Autodesk Fusion 360 part; units mm, degrees
(part 2 of 3)
  line L411 (91.783, -75.7587) -> (82.1412, -64.2681)
  line L412 (106.6546, -43.6989) -> (116.2964, -55.1895)
  line L413 (116.2964, -55.1895) -> (104.8058, -64.8313)
  line L414 (104.8058, -64.8313) -> (95.164, -53.3407)
  line L415 (95.164, -53.3407) -> (106.6546, -43.6989)
  line L416 (6.4022, 0.3248) -> (20.3282, -16.2717)
  line L417 (20.3282, -16.2717) -> (18.7961, -17.5572)
  line L418 (18.7961, -17.5572) -> (30.3663, -31.346)
  line L419 (30.3663, -31.346) -> (25.77, -35.2028)
  line L420 (25.77, -35.2028) -> (41.1969, -53.5878)
  line L421 (41.1969, -53.5878) -> (44.2611, -51.0167)
  line L422 (44.2611, -51.0167) -> (55.8313, -64.8055)
  line L423 (55.8313, -64.8055) -> (65.0238, -57.092)
  line L424 (65.0238, -57.092) -> (76.594, -70.8808)
  line L425 (76.594, -70.8808) -> (79.6582, -68.3097)
  line L426 (79.6582, -68.3097) -> (91.2284, -82.0985)
  line L427 (91.2284, -82.0985) -> (135.6589, -44.8168)
  line L428 (135.6589, -44.8168) -> (120.232, -26.4317)
  line L429 (120.232, -26.4317) -> (117.1679, -29.0029)
  line L430 (117.1679, -29.0029) -> (105.5977, -15.2141)
  line L431 (105.5977, -15.2141) -> (96.4051, -22.9275)
  line L432 (96.4051, -22.9275) -> (84.835, -9.1387)
  line L433 (84.835, -9.1387) -> (81.7708, -11.7099)
  line L434 (81.7708, -11.7099) -> (74.0573, -2.5173)
  line L435 (74.0573, -2.5173) -> (78.6536, 1.3394)
  line L436 (78.6536, 1.3394) -> (74.1541, 6.7017)
  line L437 (74.1541, 6.7017) -> (91.7731, 21.4858)
  line L438 (91.7731, 21.4858) -> (56.8473, 63.1088)
  line L439 (56.8473, 63.1088) -> (16.3349, 82)
  line L440 (16.3349, 82) -> (-38, 82)
  line L441 (-38, 82) -> (-38, 59)
  line L442 (-38, 59) -> (-45, 59)
  line L443 (-45, 59) -> (-45, 53)
  line L444 (-45, 53) -> (-57, 53)
  line L445 (-57, 53) -> (-57, 57)
  line L446 (-57, 57) -> (-75, 57)
  line L447 (-75, 57) -> (-75, 69)
  line L448 (-75, 69) -> (-93, 69)
  line L449 (-93, 69) -> (-93, 73)
  line L450 (-93, 73) -> (-117, 73)
  line L451 (-117, 73) -> (-117, 15)
  line L452 (-117, 15) -> (-99, 15)
  line L453 (-99, 15) -> (-99, 11)
  line L454 (-99, 11) -> (-81, 11)
  line L455 (-81, 11) -> (-81, -1)
  line L456 (-81, -1) -> (-63, -1)
  line L457 (-63, -1) -> (-63, -5)
  line L458 (-63, -5) -> (-39, -5)
  line L459 (-39, -5) -> (-39, 1)
  line L460 (-39, 1) -> (-21, 1)
  line L461 (-21, 1) -> (-21, 3)
  line L462 (-21, 3) -> (0.6651, 3)
  line L463 (0.6651, 3) -> (6.4022, 0.3248)
  dimension "d150" = -0.5
  dimension "d151" = -3
extrude "Extrude16" add sketch "Sketch15" along normal blind 1 contours L160 L161 L162 L163 L164 L165 L166 L167 L168 L169 L170 L171 L172 L173 L174 L175 L176 L177 L178 L179 L180 L181 L182 L183 L184 L185 L186 L187 L188 L189 L190 L191 L192 L193 L194 L195 L196 L197 L198 L199 L200 L201 L202 L203 L204 L205 L206 L207 | L292 L293 L294 L295 L296 L297 L298 L299 L300 L301 L302 L303 L304 L305 L306 L307 L308 L309 L310 L311 L312 L313 L314 L315 L316 L317 L318 L319 L320 L321 L322 L323 L324 L325 L326 L327 L328 L329 L330 L331 L332 L333 L334 L335 L336 L337 L338 L339 | L416 L417 L418 L419 L420 L421 L422 L423 L424 L425 L426 L427 L428 L429 L430 L431 L432 L433 L434 L435 L436 L437 L438 L439 L440 L441 L442 L443 L444 L445 L446 L447 L448 L449 L450 L451 L452 L453 L454 L455 L456 L457 L458 L459 L460 L461 L462 L463
sketch "Sketch16" plane through (0, 2.3, 0) normal (0, 1, 0) x (-1, 0, 0)
  line L0 (62.672, 13.3847) -> (72.3139, 1.894)
  line L1 (72.3139, 1.894) -> (60.8232, -7.7478)
  line L2 (60.8232, -7.7478) -> (51.1814, 3.7429)
  line L3 (51.1814, 3.7429) -> (62.672, 13.3847)
  line L4 (92.0203, -32.4812) -> (101.6621, -43.9719)
  line L5 (101.6621, -43.9719) -> (90.1714, -53.6137)
  line L6 (90.1714, -53.6137) -> (80.5296, -42.123)
  line L7 (80.5296, -42.123) -> (92.0203, -32.4812)
  line L8 (32.1098, -35.7574) -> (43.6004, -26.1156)
  line L9 (43.6004, -26.1156) -> (53.2423, -37.6063)
  line L10 (53.2423, -37.6063) -> (41.7516, -47.2481)
  line L11 (41.7516, -47.2481) -> (32.1098, -35.7574)
  line L12 (-58.5, 33.5) -> (-58.5, 48.5)
  line L13 (-58.5, 48.5) -> (-43.5, 48.5)
  line L14 (-43.5, 48.5) -> (-43.5, 33.5)
  line L15 (-43.5, 33.5) -> (-58.5, 33.5)
  line L16 (49.6493, 2.4573) -> (59.2911, -9.0334)
  line L17 (59.2911, -9.0334) -> (47.8004, -18.6752)
  line L18 (47.8004, -18.6752) -> (38.1586, -7.1845)
  line L19 (38.1586, -7.1845) -> (49.6493, 2.4573)
  line L20 (39.6112, 17.5317) -> (49.253, 6.041)
  line L21 (49.253, 6.041) -> (37.7623, -3.6008)
  line L22 (37.7623, -3.6008) -> (28.1205, 7.8899)
  line L23 (28.1205, 7.8899) -> (39.6112, 17.5317)
  line L24 (-40.5, 37.5) -> (-25.5, 37.5)
  line L25 (-25.5, 37.5) -> (-25.5, 22.5)
  line L26 (-25.5, 22.5) -> (-40.5, 22.5)
  line L27 (-40.5, 22.5) -> (-40.5, 37.5)
  line L28 (77.1487, -64.5411) -> (67.5068, -53.0504)
  line L29 (67.5068, -53.0504) -> (78.9975, -43.4086)
  line L30 (78.9975, -43.4086) -> (88.6393, -54.8993)
  line L31 (88.6393, -54.8993) -> (77.1487, -64.5411)
  line L32 (72.7896, -25.1203) -> (84.2803, -15.4785)
  line L33 (84.2803, -15.4785) -> (93.9221, -26.9691)
  line L34 (93.9221, -26.9691) -> (82.4315, -36.611)
  line L35 (82.4315, -36.611) -> (72.7896, -25.1203)
  line L36 (73.9427, 12.3986) -> (64.3009, 23.8893)
  line L37 (64.3009, 23.8893) -> (75.7916, 33.5311)
  line L38 (75.7916, 33.5311) -> (85.4334, 22.0405)
  line L39 (85.4334, 22.0405) -> (73.9427, 12.3986)
  line L40 (-58.5, 14.5) -> (-43.5, 14.5)
  line L41 (-43.5, 14.5) -> (-43.5, -0.5)
  line L42 (-43.5, -0.5) -> (-58.5, -0.5)
  line L43 (-58.5, -0.5) -> (-58.5, 14.5)
  line L44 (36.2303, -4.8864) -> (24.7396, -14.5282)
  line L45 (24.7396, -14.5282) -> (15.0978, -3.0375)
  line L46 (15.0978, -3.0375) -> (26.5884, 6.6043)
  line L47 (26.5884, 6.6043) -> (36.2303, -4.8864)
  line L48 (-79.5, 49.5) -> (-94.5, 49.5)
  line L49 (-94.5, 49.5) -> (-94.5, 64.5)
  line L50 (-94.5, 64.5) -> (-79.5, 64.5)
  line L51 (-79.5, 64.5) -> (-79.5, 49.5)
  line L52 (-94.5, 30.5) -> (-79.5, 30.5)
  line L53 (-79.5, 30.5) -> (-79.5, 15.5)
  line L54 (-79.5, 15.5) -> (-94.5, 15.5)
  line L55 (-94.5, 15.5) -> (-94.5, 30.5)
  line L56 (45.1325, -24.83) -> (56.6232, -15.1882)
  line L57 (56.6232, -15.1882) -> (66.265, -26.6789)
  line L58 (66.265, -26.6789) -> (54.7743, -36.3207)
  line L59 (54.7743, -36.3207) -> (45.1325, -24.83)
  line L60 (-112.5, 51.5) -> (-97.5, 51.5)
  line L61 (-97.5, 51.5) -> (-97.5, 36.5)
  line L62 (-97.5, 36.5) -> (-112.5, 36.5)
  line L63 (-112.5, 36.5) -> (-112.5, 51.5)
  line L64 (-22.5, 39.5) -> (-7.5, 39.5)
  line L65 (-7.5, 39.5) -> (-7.5, 24.5)
  line L66 (-7.5, 24.5) -> (-22.5, 24.5)
  line L67 (-22.5, 24.5) -> (-22.5, 39.5)
  line L68 (105.043, -21.5538) -> (114.6848, -33.0445)
  line L69 (114.6848, -33.0445) -> (103.1942, -42.6863)
  line L70 (103.1942, -42.6863) -> (93.5524, -31.1956)
  line L71 (93.5524, -31.1956) -> (105.043, -21.5538)
  line L72 (-15.5, 62.5) -> (-15.5, 77.5)
  line L73 (-15.5, 77.5) -> (-0.5, 77.5)
  line L74 (-0.5, 77.5) -> (-0.5, 62.5)
  line L75 (-0.5, 62.5) -> (-15.5, 62.5)
  line L76 (-40.5, 5.5) -> (-40.5, 20.5)
  line L77 (-40.5, 20.5) -> (-25.5, 20.5)
  line L78 (-25.5, 20.5) -> (-25.5, 5.5)
  line L79 (-25.5, 5.5) -> (-40.5, 5.5)
  line L80 (-58.5, 31.5) -> (-43.5, 31.5)
  line L81 (-43.5, 31.5) -> (-43.5, 16.5)
  line L82 (-43.5, 16.5) -> (-58.5, 16.5)
  line L83 (-58.5, 16.5) -> (-58.5, 31.5)
  line L84 (-22.5, 56.5) -> (-7.5, 56.5)
  line L85 (-7.5, 56.5) -> (-7.5, 41.5)
  line L86 (-7.5, 41.5) -> (-22.5, 41.5)
  line L87 (-22.5, 41.5) -> (-22.5, 56.5)
  line L88 (-61.5, 52.5) -> (-61.5, 37.5)
  line L89 (-61.5, 37.5) -> (-76.5, 37.5)
  line L90 (-76.5, 37.5) -> (-76.5, 52.5)
  line L91 (-76.5, 52.5) -> (-61.5, 52.5)
  line L92 (119.6774, -32.7715) -> (129.3192, -44.2621)
  line L93 (129.3192, -44.2621) -> (117.8285, -53.904)
  line L94 (117.8285, -53.904) -> (108.1867, -42.4133)
  line L95 (108.1867, -42.4133) -> (119.6774, -32.7715)
  line L96 (-79.5, 47.5) -> (-79.5, 32.5)
  line L97 (-79.5, 32.5) -> (-94.5, 32.5)
  line L98 (-94.5, 32.5) -> (-94.5, 47.5)
  line L99 (-94.5, 47.5) -> (-79.5, 47.5)
  line L100 (-112.5, 19.5) -> (-112.5, 34.5)
  line L101 (-112.5, 34.5) -> (-97.5, 34.5)
  line L102 (-97.5, 34.5) -> (-97.5, 19.5)
  line L103 (-97.5, 19.5) -> (-112.5, 19.5)
  line L104 (79.2878, -15.7515) -> (67.7971, -25.3933)
  line L105 (67.7971, -25.3933) -> (58.1553, -13.9026)
  line L106 (58.1553, -13.9026) -> (69.646, -4.2608)
  line L107 (69.646, -4.2608) -> (79.2878, -15.7515)
  line L108 (-76.5, 35.5) -> (-61.5, 35.5)
  line L109 (-61.5, 35.5) -> (-61.5, 20.5)
  line L110 (-61.5, 20.5) -> (-76.5, 20.5)
  line L111 (-76.5, 20.5) -> (-76.5, 35.5)
  line L112 (69.4087, -47.5383) -> (59.7669, -36.0477)
  line L113 (59.7669, -36.0477) -> (71.2576, -26.4059)
  line L114 (71.2576, -26.4059) -> (80.8994, -37.8965)
  line L115 (80.8994, -37.8965) -> (69.4087, -47.5383)
  line L116 (-112.5, 68.5) -> (-97.5, 68.5)
  line L117 (-97.5, 68.5) -> (-97.5, 53.5)
  line L118 (-97.5, 53.5) -> (-112.5, 53.5)
  line L119 (-112.5, 53.5) -> (-112.5, 68.5)
  line L120 (-25.5, 54.5) -> (-25.5, 39.5)
  line L121 (-25.5, 39.5) -> (-40.5, 39.5)
  line L122 (-40.5, 39.5) -> (-40.5, 54.5)
  line L123 (-40.5, 54.5) -> (-25.5, 54.5)
  line L124 (25.1359, -18.1119) -> (36.6265, -8.4701)
  line L125 (36.6265, -8.4701) -> (46.2683, -19.9607)
  line L126 (46.2683, -19.9607) -> (34.7777, -29.6026)
  line L127 (34.7777, -29.6026) -> (25.1359, -18.1119)
  line L128 (73.8632, 35.8293) -> (62.3725, 26.1874)
  line L129 (62.3725, 26.1874) -> (52.7307, 37.6781)
  line L130 (52.7307, 37.6781) -> (64.2214, 47.3199)
  line L131 (64.2214, 47.3199) -> (73.8632, 35.8293)
  line L132 (-76.5, 18.5) -> (-61.5, 18.5)
  line L133 (-61.5, 18.5) -> (-61.5, 3.5)
  line L134 (-61.5, 3.5) -> (-76.5, 3.5)
  line L135 (-76.5, 3.5) -> (-76.5, 18.5)
  line L136 (-33.5, 62.5) -> (-33.5, 77.5)
  line L137 (-33.5, 77.5) -> (-18.5, 77.5)
  line L138 (-18.5, 77.5) -> (-18.5, 62.5)
  line L139 (-18.5, 62.5) -> (-33.5, 62.5)
  line L140 (46.7441, -46.9751) -> (58.2348, -37.3333)
  line L141 (58.2348, -37.3333) -> (67.8766, -48.8239)
  line L142 (67.8766, -48.8239) -> (56.3859, -58.4657)
  line L143 (56.3859, -58.4657) -> (46.7441, -46.9751)
  line L144 (104.8058, -64.8313) -> (95.164, -53.3407)
  line L145 (95.164, -53.3407) -> (106.6546, -43.6989)
  line L146 (106.6546, -43.6989) -> (116.2964, -55.1895)
  line L147 (116.2964, -55.1895) -> (104.8058, -64.8313)
  line L148 (41.1433, 18.8173) -> (52.634, 28.4591)
  line L149 (52.634, 28.4591) -> (62.2758, 16.9684)
  line L150 (62.2758, 16.9684) -> (50.7851, 7.3266)
  line L151 (50.7851, 7.3266) -> (41.1433, 18.8173)
  line L152 (103.2737, -66.1169) -> (91.783, -75.7587)
  line L153 (91.783, -75.7587) -> (82.1412, -64.2681)
  line L154 (82.1412, -64.2681) -> (93.6319, -54.6263)
  line L155 (93.6319, -54.6263) -> (103.2737, -66.1169)
  line L156 (-22.5, 22.5) -> (-7.5, 22.5)
  line L157 (-7.5, 22.5) -> (-7.5, 7.5)
  line L158 (-7.5, 7.5) -> (-22.5, 7.5)
  line L159 (-22.5, 7.5) -> (-22.5, 22.5)
  line L160 (40.8272, -57.8143) -> (43.8913, -55.2432)
  line L161 (43.8913, -55.2432) -> (55.4615, -69.032)
  line L162 (55.4615, -69.032) -> (64.6541, -61.3185)
  line L163 (64.6541, -61.3185) -> (76.2242, -75.1073)
  line L164 (76.2242, -75.1073) -> (79.2884, -72.5362)
  line L165 (79.2884, -72.5362) -> (90.8586, -86.325)
  line L166 (90.8586, -86.325) -> (139.8854, -45.1866)
  line L167 (139.8854, -45.1866) -> (120.6018, -22.2052)
  line L168 (120.6018, -22.2052) -> (117.5376, -24.7764)
  line L169 (117.5376, -24.7764) -> (105.9674, -10.9876)
  line L170 (105.9674, -10.9876) -> (96.7749, -18.701)
  line L171 (96.7749, -18.701) -> (85.2047, -4.9122)
  line L172 (85.2047, -4.9122) -> (82.1406, -7.4834)
  line L173 (82.1406, -7.4834) -> (78.2838, -2.8871)
  line L174 (78.2838, -2.8871) -> (82.8801, 0.9696)
  line L175 (82.8801, 0.9696) -> (78.3806, 6.3319)
  line L176 (78.3806, 6.3319) -> (95.9996, 21.116)
  line L177 (95.9996, 21.116) -> (58.7179, 65.5466)
  line L178 (58.7179, 65.5466) -> (17, 85)
  line L179 (17, 85) -> (-41, 85)
  line L180 (-41, 85) -> (-41, 62)
  line L181 (-41, 62) -> (-48, 62)
  line L182 (-48, 62) -> (-48, 56)
  line L183 (-48, 56) -> (-54, 56)
  line L184 (-54, 56) -> (-54, 60)
  line L185 (-54, 60) -> (-72, 60)
  line L186 (-72, 60) -> (-72, 72)
  line L187 (-72, 72) -> (-90, 72)
  line L188 (-90, 72) -> (-90, 76)
  line L189 (-90, 76) -> (-120, 76)
  line L190 (-120, 76) -> (-120, 12)
  line L191 (-120, 12) -> (-102, 12)
  line L192 (-102, 12) -> (-102, 8)
  line L193 (-102, 8) -> (-84, 8)
  line L194 (-84, 8) -> (-84, -4)
  line L195 (-84, -4) -> (-66, -4)
  line L196 (-66, -4) -> (-66, -8)
  line L197 (-66, -8) -> (-36, -8)
  line L198 (-36, -8) -> (-36, -2)
  line L199 (-36, -2) -> (-18, -2)
  line L200 (-18, -2) -> (-18, 0)
  line L201 (-18, 0) -> (0, 0)
  line L202 (0, 0) -> (4.5315, -2.1131)
  line L203 (4.5315, -2.1131) -> (16.1017, -15.9019)
  line L204 (16.1017, -15.9019) -> (14.5696, -17.1875)
  line L205 (14.5696, -17.1875) -> (26.1398, -30.9763)
  line L206 (26.1398, -30.9763) -> (21.5435, -34.833)
  line L207 (21.5435, -34.833) -> (40.8272, -57.8143)
  line L208 (19.6238, -16.21) -> (18.0917, -17.4956)
  line L209 (18.0917, -17.4956) -> (29.6619, -31.2844)
  line L210 (29.6619, -31.2844) -> (25.0656, -35.1411)
  line L211 (25.0656, -35.1411) -> (41.1353, -54.2922)
  line L212 (41.1353, -54.2922) -> (44.1995, -51.7211)
  line L213 (44.1995, -51.7211) -> (55.7697, -65.5099)
  line L214 (55.7697, -65.5099) -> (64.9622, -57.7964)
  line L215 (64.9622, -57.7964) -> (76.5324, -71.5852)
  line L216 (76.5324, -71.5852) -> (79.5966, -69.0141)
  line L217 (79.5966, -69.0141) -> (91.1667, -82.8029)
  line L218 (91.1667, -82.8029) -> (136.3634, -44.8784)
  line L219 (136.3634, -44.8784) -> (120.2937, -25.7273)
  line L220 (120.2937, -25.7273) -> (117.2295, -28.2985)
  line L221 (117.2295, -28.2985) -> (105.6593, -14.5097)
  line L222 (105.6593, -14.5097) -> (96.4668, -22.2231)
  line L223 (96.4668, -22.2231) -> (84.8966, -8.4343)
  line L224 (84.8966, -8.4343) -> (81.8324, -11.0055)
  line L225 (81.8324, -11.0055) -> (74.7618, -2.579)
  line L226 (74.7618, -2.579) -> (79.358, 1.2777)
  line L227 (79.358, 1.2777) -> (74.8585, 6.6401)
  line L228 (74.8585, 6.6401) -> (92.4775, 21.4242)
  line L229 (92.4775, 21.4242) -> (57.1591, 63.5151)
  line L230 (57.1591, 63.5151) -> (16.4458, 82.5)
  line L231 (16.4458, 82.5) -> (-38.5, 82.5)
  line L232 (-38.5, 82.5) -> (-38.5, 59.5)
  line L233 (-38.5, 59.5) -> (-45.5, 59.5)
  line L234 (-45.5, 59.5) -> (-45.5, 53.5)
  line L235 (-45.5, 53.5) -> (-56.5, 53.5)
  line L236 (-56.5, 53.5) -> (-56.5, 57.5)
  line L237 (-56.5, 57.5) -> (-74.5, 57.5)
  line L238 (-74.5, 57.5) -> (-74.5, 69.5)
  line L239 (-74.5, 69.5) -> (-92.5, 69.5)
  line L240 (-92.5, 69.5) -> (-92.5, 73.5)
  line L241 (-92.5, 73.5) -> (-117.5, 73.5)
  line L242 (-117.5, 73.5) -> (-117.5, 14.5)
  line L243 (-117.5, 14.5) -> (-99.5, 14.5)
  line L244 (-99.5, 14.5) -> (-99.5, 10.5)
  line L245 (-99.5, 10.5) -> (-81.5, 10.5)
  line L246 (-81.5, 10.5) -> (-81.5, -1.5)
  line L247 (-81.5, -1.5) -> (-63.5, -1.5)
  line L248 (-63.5, -1.5) -> (-63.5, -5.5)
  line L249 (-63.5, -5.5) -> (-38.5, -5.5)
  line L250 (-38.5, -5.5) -> (-38.5, 0.5)
  line L251 (-38.5, 0.5) -> (-20.5, 0.5)
  line L252 (-20.5, 0.5) -> (-20.5, 2.5)
  line L253 (-20.5, 2.5) -> (0.5542, 2.5)
  line L254 (0.5542, 2.5) -> (6.0904, -0.0816)
  line L255 (6.0904, -0.0816) -> (19.6238, -16.21)
  dimension "d154" = -2.5
extrude "Extrude17" add sketch "Sketch16" along normal blind 4.7 contours L160 L161 L162 L163 L164 L165 L166 L167 L168 L169 L170 L171 L172 L173 L174 L175 L176 L177 L178 L179 L180 L181 L182 L183 L184 L185 L186 L187 L188 L189 L190 L191 L192 L193 L194 L195 L196 L197 L198 L199 L200 L201 L202 L203 L204 L205 L206 L207
sketch "Sketch18" plane through (0, 7, 0) normal (0, 1, 0) x (-1, 0, 0)
  line L0 (19.6238, -16.21) -> (6.0904, -0.0816)
  line L1 (6.0904, -0.0816) -> (0.5542, 2.5)
  line L2 (0.5542, 2.5) -> (-20.5, 2.5)
  line L3 (-20.5, 2.5) -> (-20.5, 0.5)
  line L4 (-20.5, 0.5) -> (-38.5, 0.5)
  line L5 (-38.5, 0.5) -> (-38.5, -5.5)
  line L6 (-38.5, -5.5) -> (-63.5, -5.5)
  line L7 (-63.5, -5.5) -> (-63.5, -1.5)
  line L8 (-63.5, -1.5) -> (-81.5, -1.5)
  line L9 (-81.5, -1.5) -> (-81.5, 10.5)
  line L10 (-81.5, 10.5) -> (-99.5, 10.5)
  line L11 (-99.5, 10.5) -> (-99.5, 14.5)
  line L12 (-99.5, 14.5) -> (-117.5, 14.5)
  line L13 (-117.5, 14.5) -> (-117.5, 73.5)
  line L14 (-117.5, 73.5) -> (-92.5, 73.5)
  line L15 (-92.5, 73.5) -> (-92.5, 69.5)
  line L16 (-92.5, 69.5) -> (-74.5, 69.5)
  line L17 (-74.5, 69.5) -> (-74.5, 57.5)
  line L18 (-74.5, 57.5) -> (-56.5, 57.5)
  line L19 (-56.5, 57.5) -> (-56.5, 53.5)
  line L20 (-56.5, 53.5) -> (-45.5, 53.5)
  line L21 (-45.5, 53.5) -> (-45.5, 59.5)
  line L22 (-45.5, 59.5) -> (-38.5, 59.5)
  line L23 (-38.5, 59.5) -> (-38.5, 82.5)
  line L24 (-38.5, 82.5) -> (16.4458, 82.5)
  line L25 (16.4458, 82.5) -> (57.1591, 63.5151)
  line L26 (57.1591, 63.5151) -> (92.4775, 21.4242)
  line L27 (92.4775, 21.4242) -> (74.8585, 6.6401)
  line L28 (74.8585, 6.6401) -> (79.358, 1.2777)
  line L29 (79.358, 1.2777) -> (74.7618, -2.579)
  line L30 (74.7618, -2.579) -> (81.8324, -11.0055)
  line L31 (81.8324, -11.0055) -> (84.8966, -8.4343)
  line L32 (84.8966, -8.4343) -> (96.4668, -22.2231)
  line L33 (96.4668, -22.2231) -> (105.6593, -14.5097)
  line L34 (105.6593, -14.5097) -> (117.2295, -28.2985)
  line L35 (117.2295, -28.2985) -> (120.2937, -25.7273)
  line L36 (120.2937, -25.7273) -> (136.3634, -44.8784)
  line L37 (136.3634, -44.8784) -> (91.1667, -82.8029)
  line L38 (91.1667, -82.8029) -> (79.5966, -69.0141)
  line L39 (79.5966, -69.0141) -> (76.5324, -71.5852)
  line L40 (76.5324, -71.5852) -> (64.9622, -57.7964)
  line L41 (64.9622, -57.7964) -> (55.7697, -65.5099)
  line L42 (55.7697, -65.5099) -> (44.1995, -51.7211)
  line L43 (44.1995, -51.7211) -> (41.1353, -54.2922)
  line L44 (41.1353, -54.2922) -> (25.0656, -35.1411)
  line L45 (25.0656, -35.1411) -> (29.6619, -31.2844)
  line L46 (29.6619, -31.2844) -> (18.0917, -17.4956)
  line L47 (18.0917, -17.4956) -> (19.6238, -16.21)
  line L48 (21.5435, -34.833) -> (40.8272, -57.8143)
  line L49 (40.8272, -57.8143) -> (43.8913, -55.2432)
  line L50 (43.8913, -55.2432) -> (55.4615, -69.032)
  line L51 (55.4615, -69.032) -> (64.6541, -61.3185)
  line L52 (64.6541, -61.3185) -> (76.2242, -75.1073)
  line L53 (76.2242, -75.1073) -> (79.2884, -72.5362)
  line L54 (79.2884, -72.5362) -> (90.8586, -86.325)
  line L55 (90.8586, -86.325) -> (139.8854, -45.1866)
  line L56 (139.8854, -45.1866) -> (120.6018, -22.2052)
  line L57 (120.6018, -22.2052) -> (117.5376, -24.7764)
  line L58 (117.5376, -24.7764) -> (105.9674, -10.9876)
  line L59 (105.9674, -10.9876) -> (96.7749, -18.701)
  line L60 (96.7749, -18.701) -> (85.2047, -4.9122)
  line L61 (85.2047, -4.9122) -> (82.1406, -7.4834)
  line L62 (82.1406, -7.4834) -> (78.2838, -2.8871)
  line L63 (78.2838, -2.8871) -> (82.8801, 0.9696)
  line L64 (82.8801, 0.9696) -> (78.3806, 6.3319)
  line L65 (78.3806, 6.3319) -> (95.9996, 21.116)
  line L66 (95.9996, 21.116) -> (58.7179, 65.5466)
  line L67 (58.7179, 65.5466) -> (17, 85)
  line L68 (17, 85) -> (-41, 85)
  line L69 (-41, 85) -> (-41, 62)
  line L70 (-41, 62) -> (-48, 62)
  line L71 (-48, 62) -> (-48, 56)
  line L72 (-48, 56) -> (-54, 56)
  line L73 (-54, 56) -> (-54, 60)
  line L74 (-54, 60) -> (-72, 60)
  line L75 (-72, 60) -> (-72, 72)
  line L76 (-72, 72) -> (-90, 72)
  line L77 (-90, 72) -> (-90, 76)
  line L78 (-90, 76) -> (-120, 76)
  line L79 (-120, 76) -> (-120, 12)
  line L80 (-120, 12) -> (-102, 12)
  line L81 (-102, 12) -> (-102, 8)
  line L82 (-102, 8) -> (-84, 8)
  line L83 (-84, 8) -> (-84, -4)
  line L84 (-84, -4) -> (-66, -4)
  line L85 (-66, -4) -> (-66, -8)
  line L86 (-66, -8) -> (-36, -8)
  line L87 (-36, -8) -> (-36, -2)
  line L88 (-36, -2) -> (-18, -2)
  line L89 (-18, -2) -> (-18, 0)
  line L90 (-18, 0) -> (0, 0)
  line L91 (0, 0) -> (4.5315, -2.1131)
  line L92 (4.5315, -2.1131) -> (16.1017, -15.9019)
  line L93 (16.1017, -15.9019) -> (14.5696, -17.1875)
  line L94 (14.5696, -17.1875) -> (26.1398, -30.9763)
  line L95 (26.1398, -30.9763) -> (21.5435, -34.833)
  line L96 (14.5696, -17.1875) -> (-18, -2)
  constraint coincident L93.end L94.start
  constraint coincident L88.end L89.start
extrude "Extrude18" add sketch "Sketch18" against normal blind 7 contours L89 L90 L91 L92 L93 L96
sketch "Sketch19" plane through (3.981, 0, -8.5372) normal (0.422618, 0, -0.906308) x (-0.906308, 0, -0.422618)
  line L0 (20.4683, 7) -> (-15.4683, 7)
  line L1 (-15.4683, 7) -> (-15.4683, 0)
  line L2 (-15.4683, 0) -> (20.4683, 0)
  line L3 (20.4683, 0) -> (20.4683, 7)
  line L4 (2.5, 7) -> (2.5, 0)
  line L5 (2.5, 7) -> (2.5, 1.3)
  line L6 (2.5, 1.3) -> (8.4, 1.3)
  line L7 (2.5, 1.3) -> (-3.4, 1.3)
  line L8 (-3.4, 1.3) -> (-3.4, 7)
  line L9 (8.4, 1.3) -> (8.4, 7)
  line L10 (8.4, 7) -> (-3.4, 7)
  line L11 (-3.4, 1.3) -> (-3.2445, 1.3)
  dimension "d161" = 5.7
  dimension "d162" = 5.9
  dimension "d163" = 5.9
  constraint midpoint L0 L4.start
  constraint midpoint L2 L4.end
  constraint perpendicular L0 L5
  constraint perpendicular L5 L6
  constraint perpendicular L4 L7
  constraint coincident L0 L8.end
  constraint perpendicular L0 L8
  constraint coincident L0 L9.end
  constraint perpendicular L0 L9
  constraint coincident L7 L11.end
  constraint perpendicular L8 L11
  measures "d161" distance of L4.start L5.end
  measures "d162" distance of L5.end L6.end
  measures "d163" distance of L5.end L7.end
extrude "Extrude19" cut sketch "Sketch19" against normal blind 12 contours L0 L4 L5 L6 L9 L10 | L0 L4 L5 L7 L8 L10 L11
fillet "Fillet4" radius 2.85 2 edges at (4.5267, 1.3, -1.6624) (-6.1677, 1.3, -6.6493)
sketch "Sketch20" plane through (0, 2.3, 0) normal (0, 1, 0) x (-1, 0, 0)
  line L0 (7.625, -1.9104) -> (19.6238, -16.21)
  line L1 (19.6238, -16.21) -> (18.0917, -17.4956)
  line L2 (18.0917, -17.4956) -> (29.6619, -31.2844)
  line L3 (29.6619, -31.2844) -> (25.0656, -35.1411)
  line L4 (25.0656, -35.1411) -> (41.1353, -54.2922)
  line L5 (41.1353, -54.2922) -> (44.1995, -51.7211)
  line L6 (44.1995, -51.7211) -> (55.7697, -65.5099)
  line L7 (55.7697, -65.5099) -> (64.9622, -57.7964)
  line L8 (64.9622, -57.7964) -> (76.5324, -71.5852)
  line L9 (76.5324, -71.5852) -> (79.5966, -69.0141)
  line L10 (79.5966, -69.0141) -> (91.1667, -82.8029)
  line L11 (91.1667, -82.8029) -> (136.3634, -44.8784)
  line L12 (136.3634, -44.8784) -> (120.2937, -25.7273)
  line L13 (120.2937, -25.7273) -> (117.2295, -28.2985)
  line L14 (117.2295, -28.2985) -> (105.6593, -14.5097)
  line L15 (105.6593, -14.5097) -> (96.4668, -22.2231)
  line L16 (96.4668, -22.2231) -> (84.8966, -8.4343)
  line L17 (84.8966, -8.4343) -> (81.8324, -11.0055)
  line L18 (81.8324, -11.0055) -> (74.7618, -2.579)
  line L19 (74.7618, -2.579) -> (79.358, 1.2777)
  line L20 (79.358, 1.2777) -> (74.8585, 6.6401)
  line L21 (74.8585, 6.6401) -> (92.4775, 21.4242)
  line L22 (92.4775, 21.4242) -> (57.1591, 63.5151)
  line L23 (57.1591, 63.5151) -> (16.4458, 82.5)
  line L24 (16.4458, 82.5) -> (-38.5, 82.5)
  line L25 (-38.5, 82.5) -> (-38.5, 59.5)
  line L26 (-38.5, 59.5) -> (-45.5, 59.5)
  line L27 (-45.5, 59.5) -> (-45.5, 53.5)
  line L28 (-45.5, 53.5) -> (-56.5, 53.5)
  line L29 (-56.5, 53.5) -> (-56.5, 57.5)
  line L30 (-56.5, 57.5) -> (-74.5, 57.5)
  line L31 (-74.5, 57.5) -> (-74.5, 69.5)
  line L32 (-74.5, 69.5) -> (-92.5, 69.5)
  line L33 (-92.5, 69.5) -> (-92.5, 73.5)
  line L34 (-92.5, 73.5) -> (-117.5, 73.5)
  line L35 (-117.5, 73.5) -> (-117.5, 14.5)
  line L36 (-117.5, 14.5) -> (-99.5, 14.5)
  line L37 (-99.5, 14.5) -> (-99.5, 10.5)
  line L38 (-99.5, 10.5) -> (-81.5, 10.5)
  line L39 (-81.5, 10.5) -> (-81.5, -1.5)
  line L40 (-81.5, -1.5) -> (-63.5, -1.5)
  line L41 (-63.5, -1.5) -> (-63.5, -5.5)
  line L42 (-63.5, -5.5) -> (-38.5, -5.5)
  line L43 (-38.5, -5.5) -> (-38.5, 0.5)
  line L44 (-38.5, 0.5) -> (-20.5, 0.5)
  line L45 (-20.5, 0.5) -> (-20.5, 2.5)
  line L46 (-20.5, 2.5) -> (-1.8332, 2.5)
  line L47 (-1.8332, 2.5) -> (-1.3728, 3.4872)
  line L48 (-1.3728, 3.4872) -> (8.0853, -0.9232)
  line L49 (8.0853, -0.9232) -> (7.625, -1.9104)
  line L50 (62.672, 13.3847) -> (72.3139, 1.894)
  line L51 (72.3139, 1.894) -> (60.8232, -7.7478)
  line L52 (60.8232, -7.7478) -> (51.1814, 3.7429)
  line L53 (51.1814, 3.7429) -> (62.672, 13.3847)
  line L54 (92.0203, -32.4812) -> (101.6621, -43.9719)
  line L55 (101.6621, -43.9719) -> (90.1714, -53.6137)
  line L56 (90.1714, -53.6137) -> (80.5296, -42.123)
  line L57 (80.5296, -42.123) -> (92.0203, -32.4812)
  line L58 (49.6493, 2.4573) -> (59.2911, -9.0334)
  line L59 (59.2911, -9.0334) -> (47.8004, -18.6752)
  line L60 (47.8004, -18.6752) -> (38.1586, -7.1845)
  line L61 (38.1586, -7.1845) -> (49.6493, 2.4573)
  line L62 (77.1487, -64.5411) -> (67.5068, -53.0504)
  line L63 (67.5068, -53.0504) -> (78.9975, -43.4086)
  line L64 (78.9975, -43.4086) -> (88.6393, -54.8993)
  line L65 (88.6393, -54.8993) -> (77.1487, -64.5411)
  line L66 (-40.5, 37.5) -> (-25.5, 37.5)
  line L67 (-25.5, 37.5) -> (-25.5, 22.5)
  line L68 (-25.5, 22.5) -> (-40.5, 22.5)
  line L69 (-40.5, 22.5) -> (-40.5, 37.5)
  line L70 (32.1098, -35.7574) -> (43.6004, -26.1156)
  line L71 (43.6004, -26.1156) -> (53.2423, -37.6063)
  line L72 (53.2423, -37.6063) -> (41.7516, -47.2481)
  line L73 (41.7516, -47.2481) -> (32.1098, -35.7574)
  line L74 (69.4087, -47.5383) -> (59.7669, -36.0477)
  line L75 (59.7669, -36.0477) -> (71.2576, -26.4059)
  line L76 (71.2576, -26.4059) -> (80.8994, -37.8965)
  line L77 (80.8994, -37.8965) -> (69.4087, -47.5383)
  line L78 (39.6112, 17.5317) -> (49.253, 6.041)
  line L79 (49.253, 6.041) -> (37.7623, -3.6008)
  line L80 (37.7623, -3.6008) -> (28.1205, 7.8899)
  line L81 (28.1205, 7.8899) -> (39.6112, 17.5317)
  line L82 (-58.5, 33.5) -> (-58.5, 48.5)
  line L83 (-58.5, 48.5) -> (-43.5, 48.5)
  line L84 (-43.5, 48.5) -> (-43.5, 33.5)
  line L85 (-43.5, 33.5) -> (-58.5, 33.5)
  line L86 (119.6774, -32.7715) -> (129.3192, -44.2621)
  line L87 (129.3192, -44.2621) -> (117.8285, -53.904)
  line L88 (117.8285, -53.904) -> (108.1867, -42.4133)
  line L89 (108.1867, -42.4133) -> (119.6774, -32.7715)
  line L90 (-76.5, 18.5) -> (-61.5, 18.5)
  line L91 (-61.5, 18.5) -> (-61.5, 3.5)
  line L92 (-61.5, 3.5) -> (-76.5, 3.5)
  line L93 (-76.5, 3.5) -> (-76.5, 18.5)
  line L94 (73.8632, 35.8293) -> (62.3725, 26.1874)
  line L95 (62.3725, 26.1874) -> (52.7307, 37.6781)
  line L96 (52.7307, 37.6781) -> (64.2214, 47.3199)
  line L97 (64.2214, 47.3199) -> (73.8632, 35.8293)
  line L98 (25.1359, -18.1119) -> (36.6265, -8.4701)
  line L99 (36.6265, -8.4701) -> (46.2683, -19.9607)
  line L100 (46.2683, -19.9607) -> (34.7777, -29.6026)
  line L101 (34.7777, -29.6026) -> (25.1359, -18.1119)
  line L102 (-94.5, 30.5) -> (-79.5, 30.5)
  line L103 (-79.5, 30.5) -> (-79.5, 15.5)
  line L104 (-79.5, 15.5) -> (-94.5, 15.5)
  line L105 (-94.5, 15.5) -> (-94.5, 30.5)
  line L106 (45.1325, -24.83) -> (56.6232, -15.1882)
  line L107 (56.6232, -15.1882) -> (66.265, -26.6789)
  line L108 (66.265, -26.6789) -> (54.7743, -36.3207)
  line L109 (54.7743, -36.3207) -> (45.1325, -24.83)
  line L110 (-112.5, 51.5) -> (-97.5, 51.5)
  line L111 (-97.5, 51.5) -> (-97.5, 36.5)
  line L112 (-97.5, 36.5) -> (-112.5, 36.5)
  line L113 (-112.5, 36.5) -> (-112.5, 51.5)
  line L114 (-22.5, 39.5) -> (-7.5, 39.5)
  line L115 (-7.5, 39.5) -> (-7.5, 24.5)
  line L116 (-7.5, 24.5) -> (-22.5, 24.5)
  line L117 (-22.5, 24.5) -> (-22.5, 39.5)
  line L118 (105.043, -21.5538) -> (114.6848, -33.0445)
  line L119 (114.6848, -33.0445) -> (103.1942, -42.6863)
  line L120 (103.1942, -42.6863) -> (93.5524, -31.1956)
  line L121 (93.5524, -31.1956) -> (105.043, -21.5538)
  line L122 (-15.5, 62.5) -> (-15.5, 77.5)
  line L123 (-15.5, 77.5) -> (-0.5, 77.5)
  line L124 (-0.5, 77.5) -> (-0.5, 62.5)
  line L125 (-0.5, 62.5) -> (-15.5, 62.5)
  line L126 (-40.5, 5.5) -> (-40.5, 20.5)
  line L127 (-40.5, 20.5) -> (-25.5, 20.5)
  line L128 (-25.5, 20.5) -> (-25.5, 5.5)
  line L129 (-25.5, 5.5) -> (-40.5, 5.5)
  line L130 (-58.5, 31.5) -> (-43.5, 31.5)
  line L131 (-43.5, 31.5) -> (-43.5, 16.5)
  line L132 (-43.5, 16.5) -> (-58.5, 16.5)
  line L133 (-58.5, 16.5) -> (-58.5, 31.5)
  line L134 (-22.5, 56.5) -> (-7.5, 56.5)
  line L135 (-7.5, 56.5) -> (-7.5, 41.5)
  line L136 (-7.5, 41.5) -> (-22.5, 41.5)
  line L137 (-22.5, 41.5) -> (-22.5, 56.5)
  line L138 (72.7896, -25.1203) -> (84.2803, -15.4785)
  line L139 (84.2803, -15.4785) -> (93.9221, -26.9691)
  line L140 (93.9221, -26.9691) -> (82.4315, -36.611)
  line L141 (82.4315, -36.611) -> (72.7896, -25.1203)
  line L142 (103.2737, -66.1169) -> (91.783, -75.7587)
  line L143 (91.783, -75.7587) -> (82.1412, -64.2681)
  line L144 (82.1412, -64.2681) -> (93.6319, -54.6263)
  line L145 (93.6319, -54.6263) -> (103.2737, -66.1169)
  line L146 (-33.5, 62.5) -> (-33.5, 77.5)
  line L147 (-33.5, 77.5) -> (-18.5, 77.5)
  line L148 (-18.5, 77.5) -> (-18.5, 62.5)
  line L149 (-18.5, 62.5) -> (-33.5, 62.5)
  line L150 (46.7441, -46.9751) -> (58.2348, -37.3333)
  line L151 (58.2348, -37.3333) -> (67.8766, -48.8239)
  line L152 (67.8766, -48.8239) -> (56.3859, -58.4657)
  line L153 (56.3859, -58.4657) -> (46.7441, -46.9751)
  line L154 (-22.5, 22.5) -> (-7.5, 22.5)
  line L155 (-7.5, 22.5) -> (-7.5, 7.5)
  line L156 (-7.5, 7.5) -> (-22.5, 7.5)
  line L157 (-22.5, 7.5) -> (-22.5, 22.5)
  line L158 (41.1433, 18.8173) -> (52.634, 28.4591)
  line L159 (52.634, 28.4591) -> (62.2758, 16.9684)
  line L160 (62.2758, 16.9684) -> (50.7851, 7.3266)
  line L161 (50.7851, 7.3266) -> (41.1433, 18.8173)
  line L162 (73.9427, 12.3986) -> (64.3009, 23.8893)
  line L163 (64.3009, 23.8893) -> (75.7916, 33.5311)
  line L164 (75.7916, 33.5311) -> (85.4334, 22.0405)
  line L165 (85.4334, 22.0405) -> (73.9427, 12.3986)
  line L166 (-61.5, 52.5) -> (-61.5, 37.5)
  line L167 (-61.5, 37.5) -> (-76.5, 37.5)
  line L168 (-76.5, 37.5) -> (-76.5, 52.5)
  line L169 (-76.5, 52.5) -> (-61.5, 52.5)
  line L170 (-79.5, 49.5) -> (-94.5, 49.5)
  line L171 (-94.5, 49.5) -> (-94.5, 64.5)
  line L172 (-94.5, 64.5) -> (-79.5, 64.5)
  line L173 (-79.5, 64.5) -> (-79.5, 49.5)
  line L174 (-25.5, 54.5) -> (-25.5, 39.5)
  line L175 (-25.5, 39.5) -> (-40.5, 39.5)
  line L176 (-40.5, 39.5) -> (-40.5, 54.5)
  line L177 (-40.5, 54.5) -> (-25.5, 54.5)
  line L178 (-79.5, 47.5) -> (-79.5, 32.5)
  line L179 (-79.5, 32.5) -> (-94.5, 32.5)
  line L180 (-94.5, 32.5) -> (-94.5, 47.5)
  line L181 (-94.5, 47.5) -> (-79.5, 47.5)
  line L182 (-112.5, 19.5) -> (-112.5, 34.5)
  line L183 (-112.5, 34.5) -> (-97.5, 34.5)
  line L184 (-97.5, 34.5) -> (-97.5, 19.5)
  line L185 (-97.5, 19.5) -> (-112.5, 19.5)
  line L186 (36.2303, -4.8864) -> (24.7396, -14.5282)
  line L187 (24.7396, -14.5282) -> (15.0978, -3.0375)
  line L188 (15.0978, -3.0375) -> (26.5884, 6.6043)
  line L189 (26.5884, 6.6043) -> (36.2303, -4.8864)
  line L190 (79.2878, -15.7515) -> (67.7971, -25.3933)
  line L191 (67.7971, -25.3933) -> (58.1553, -13.9026)
  line L192 (58.1553, -13.9026) -> (69.646, -4.2608)
  line L193 (69.646, -4.2608) -> (79.2878, -15.7515)
  line L194 (-58.5, 14.5) -> (-43.5, 14.5)
  line L195 (-43.5, 14.5) -> (-43.5, -0.5)
  line L196 (-43.5, -0.5) -> (-58.5, -0.5)
  line L197 (-58.5, -0.5) -> (-58.5, 14.5)
  line L198 (-76.5, 35.5) -> (-61.5, 35.5)
  line L199 (-61.5, 35.5) -> (-61.5, 20.5)
  line L200 (-61.5, 20.5) -> (-76.5, 20.5)
  line L201 (-76.5, 20.5) -> (-76.5, 35.5)
  line L202 (-112.5, 68.5) -> (-97.5, 68.5)
  line L203 (-97.5, 68.5) -> (-97.5, 53.5)
  line L204 (-97.5, 53.5) -> (-112.5, 53.5)
  line L205 (-112.5, 53.5) -> (-112.5, 68.5)
  line L206 (104.8058, -64.8313) -> (95.164, -53.3407)
  line L207 (95.164, -53.3407) -> (106.6546, -43.6989)
  line L208 (106.6546, -43.6989) -> (116.2964, -55.1895)
  line L209 (116.2964, -55.1895) -> (104.8058, -64.8313)
  line L210 (3.3562, 1.282) -> (36.8024, 73.0075)
  line L211 (3.3562, 1.282) -> (3.7789, 2.1883)
  line L212 (3.7789, 2.1883) -> (-4.3779, 5.9918)
  line L213 (3.7789, 2.1883) -> (11.9356, -1.6153)
  line L214 (11.9356, -1.6153) -> (-4.3779, 5.9918)
  line L215 (-4.3779, 5.9918) -> (10.4137, 37.7126)
  line L216 (10.4137, 37.7126) -> (26.7273, 30.1055)
  line L217 (26.7273, 30.1055) -> (11.9356, -1.6153)
  dimension "d168" = 1
  dimension "d169" = 9
  dimension "d170" = 9
  dimension "d171" = 35
  constraint midpoint L48 L210.start
  constraint midpoint L23 L210.end
  constraint perpendicular L48 L211
  constraint perpendicular L211 L212
  constraint perpendicular L211 L213
  constraint perpendicular L214 L215
  constraint parallel L214 L216
  constraint parallel L215 L217
  measures "d168" distance of L210.start L211.end
  measures "d169" distance of L211.end L212.end
  measures "d170" distance of L211.end L213.end
  measures "d171" distance of L213.end L216.end
extrude "Extrude20" cut sketch "Sketch20" against normal blind 2 contours L210 L212 L214 L215 L216 | L210 L213 L214 L216 L217
sketch "Sketch21" plane through (0, 2.3, 0) normal (0, 1, 0) x (-1, 0, 0)
  line L0 (-4.3779, 5.9918) -> (10.4137, 37.7126)
  line L1 (10.4137, 37.7126) -> (26.7273, 30.1055)
  line L2 (26.7273, 30.1055) -> (11.9356, -1.6153)
  line L3 (11.9356, -1.6153) -> (-4.3779, 5.9918)
  line L4 (7.625, -1.9104) -> (19.6238, -16.21)
  line L5 (19.6238, -16.21) -> (18.0917, -17.4956)
  line L6 (18.0917, -17.4956) -> (29.6619, -31.2844)
  line L7 (29.6619, -31.2844) -> (25.0656, -35.1411)
  line L8 (25.0656, -35.1411) -> (41.1353, -54.2922)
  line L9 (41.1353, -54.2922) -> (44.1995, -51.7211)
  line L10 (44.1995, -51.7211) -> (55.7697, -65.5099)
  line L11 (55.7697, -65.5099) -> (64.9622, -57.7964)
  line L12 (64.9622, -57.7964) -> (76.5324, -71.5852)
  line L13 (76.5324, -71.5852) -> (79.5966, -69.0141)
  line L14 (79.5966, -69.0141) -> (91.1667, -82.8029)
  line L15 (91.1667, -82.8029) -> (136.3634, -44.8784)
  line L16 (136.3634, -44.8784) -> (120.2937, -25.7273)
  line L17 (120.2937, -25.7273) -> (117.2295, -28.2985)
  line L18 (117.2295, -28.2985) -> (105.6593, -14.5097)
  line L19 (105.6593, -14.5097) -> (96.4668, -22.2231)
  line L20 (96.4668, -22.2231) -> (84.8966, -8.4343)
  line L21 (84.8966, -8.4343) -> (81.8324, -11.0055)
  line L22 (81.8324, -11.0055) -> (74.7618, -2.579)
  line L23 (74.7618, -2.579) -> (79.358, 1.2777)
  line L24 (79.358, 1.2777) -> (74.8585, 6.6401)
  line L25 (74.8585, 6.6401) -> (92.4775, 21.4242)
  line L26 (92.4775, 21.4242) -> (57.1591, 63.5151)
  line L27 (57.1591, 63.5151) -> (16.4458, 82.5)
  line L28 (16.4458, 82.5) -> (-38.5, 82.5)
  line L29 (-38.5, 82.5) -> (-38.5, 59.5)
  line L30 (-38.5, 59.5) -> (-45.5, 59.5)
  line L31 (-45.5, 59.5) -> (-45.5, 53.5)
  line L32 (-45.5, 53.5) -> (-56.5, 53.5)
  line L33 (-56.5, 53.5) -> (-56.5, 57.5)
  line L34 (-56.5, 57.5) -> (-74.5, 57.5)
  line L35 (-74.5, 57.5) -> (-74.5, 69.5)
  line L36 (-74.5, 69.5) -> (-92.5, 69.5)
  line L37 (-92.5, 69.5) -> (-92.5, 73.5)
  line L38 (-92.5, 73.5) -> (-117.5, 73.5)
  line L39 (-117.5, 73.5) -> (-117.5, 14.5)
  line L40 (-117.5, 14.5) -> (-99.5, 14.5)
  line L41 (-99.5, 14.5) -> (-99.5, 10.5)
  line L42 (-99.5, 10.5) -> (-81.5, 10.5)
  line L43 (-81.5, 10.5) -> (-81.5, -1.5)
  line L44 (-81.5, -1.5) -> (-63.5, -1.5)
  line L45 (-63.5, -1.5) -> (-63.5, -5.5)
  line L46 (-63.5, -5.5) -> (-38.5, -5.5)
  line L47 (-38.5, -5.5) -> (-38.5, 0.5)
  line L48 (-38.5, 0.5) -> (-20.5, 0.5)
  line L49 (-20.5, 0.5) -> (-20.5, 2.5)
  line L50 (-20.5, 2.5) -> (-1.8332, 2.5)
  line L51 (-1.8332, 2.5) -> (-1.3728, 3.4872)
  line L52 (-1.3728, 3.4872) -> (8.0853, -0.9232)
  line L53 (8.0853, -0.9232) -> (7.625, -1.9104)
  line L54 (62.672, 13.3847) -> (72.3139, 1.894)
  line L55 (72.3139, 1.894) -> (60.8232, -7.7478)
  line L56 (60.8232, -7.7478) -> (51.1814, 3.7429)
  line L57 (51.1814, 3.7429) -> (62.672, 13.3847)
  line L58 (92.0203, -32.4812) -> (101.6621, -43.9719)
  line L59 (101.6621, -43.9719) -> (90.1714, -53.6137)
  line L60 (90.1714, -53.6137) -> (80.5296, -42.123)
  line L61 (80.5296, -42.123) -> (92.0203, -32.4812)
  line L62 (49.6493, 2.4573) -> (59.2911, -9.0334)
  line L63 (59.2911, -9.0334) -> (47.8004, -18.6752)
  line L64 (47.8004, -18.6752) -> (38.1586, -7.1845)
  line L65 (38.1586, -7.1845) -> (49.6493, 2.4573)
  line L66 (77.1487, -64.5411) -> (67.5068, -53.0504)
  line L67 (67.5068, -53.0504) -> (78.9975, -43.4086)
  line L68 (78.9975, -43.4086) -> (88.6393, -54.8993)
  line L69 (88.6393, -54.8993) -> (77.1487, -64.5411)
  line L70 (-40.5, 37.5) -> (-25.5, 37.5)
  line L71 (-25.5, 37.5) -> (-25.5, 22.5)
  line L72 (-25.5, 22.5) -> (-40.5, 22.5)
  line L73 (-40.5, 22.5) -> (-40.5, 37.5)
  line L74 (32.1098, -35.7574) -> (43.6004, -26.1156)
  line L75 (43.6004, -26.1156) -> (53.2423, -37.6063)
  line L76 (53.2423, -37.6063) -> (41.7516, -47.2481)
  line L77 (41.7516, -47.2481) -> (32.1098, -35.7574)
  line L78 (69.4087, -47.5383) -> (59.7669, -36.0477)
  line L79 (59.7669, -36.0477) -> (71.2576, -26.4059)
  line L80 (71.2576, -26.4059) -> (80.8994, -37.8965)
  line L81 (80.8994, -37.8965) -> (69.4087, -47.5383)
  line L82 (39.6112, 17.5317) -> (49.253, 6.041)
  line L83 (49.253, 6.041) -> (37.7623, -3.6008)
  line L84 (37.7623, -3.6008) -> (28.1205, 7.8899)
  line L85 (28.1205, 7.8899) -> (39.6112, 17.5317)
  line L86 (-58.5, 33.5) -> (-58.5, 48.5)
  line L87 (-58.5, 48.5) -> (-43.5, 48.5)
  line L88 (-43.5, 48.5) -> (-43.5, 33.5)
  line L89 (-43.5, 33.5) -> (-58.5, 33.5)
  line L90 (119.6774, -32.7715) -> (129.3192, -44.2621)
  line L91 (129.3192, -44.2621) -> (117.8285, -53.904)
  line L92 (117.8285, -53.904) -> (108.1867, -42.4133)
  line L93 (108.1867, -42.4133) -> (119.6774, -32.7715)
  line L94 (-76.5, 18.5) -> (-61.5, 18.5)
  line L95 (-61.5, 18.5) -> (-61.5, 3.5)
  line L96 (-61.5, 3.5) -> (-76.5, 3.5)
  line L97 (-76.5, 3.5) -> (-76.5, 18.5)
  line L98 (73.8632, 35.8293) -> (62.3725, 26.1874)
  line L99 (62.3725, 26.1874) -> (52.7307, 37.6781)
  line L100 (52.7307, 37.6781) -> (64.2214, 47.3199)
  line L101 (64.2214, 47.3199) -> (73.8632, 35.8293)
  line L102 (25.1359, -18.1119) -> (36.6265, -8.4701)
  line L103 (36.6265, -8.4701) -> (46.2683, -19.9607)
  line L104 (46.2683, -19.9607) -> (34.7777, -29.6026)
  line L105 (34.7777, -29.6026) -> (25.1359, -18.1119)
  line L106 (-94.5, 30.5) -> (-79.5, 30.5)
  line L107 (-79.5, 30.5) -> (-79.5, 15.5)
  line L108 (-79.5, 15.5) -> (-94.5, 15.5)
  line L109 (-94.5, 15.5) -> (-94.5, 30.5)
  line L110 (45.1325, -24.83) -> (56.6232, -15.1882)
  line L111 (56.6232, -15.1882) -> (66.265, -26.6789)
  line L112 (66.265, -26.6789) -> (54.7743, -36.3207)
  line L113 (54.7743, -36.3207) -> (45.1325, -24.83)
  line L114 (-112.5, 51.5) -> (-97.5, 51.5)
  line L115 (-97.5, 51.5) -> (-97.5, 36.5)
  line L116 (-97.5, 36.5) -> (-112.5, 36.5)
  line L117 (-112.5, 36.5) -> (-112.5, 51.5)
  line L118 (-22.5, 39.5) -> (-7.5, 39.5)
  line L119 (-7.5, 39.5) -> (-7.5, 24.5)
  line L120 (-7.5, 24.5) -> (-22.5, 24.5)
  line L121 (-22.5, 24.5) -> (-22.5, 39.5)
  line L122 (105.043, -21.5538) -> (114.6848, -33.0445)
  line L123 (114.6848, -33.0445) -> (103.1942, -42.6863)
  line L124 (103.1942, -42.6863) -> (93.5524, -31.1956)
  line L125 (93.5524, -31.1956) -> (105.043, -21.5538)
  line L126 (-15.5, 62.5) -> (-15.5, 77.5)
  line L127 (-15.5, 77.5) -> (-0.5, 77.5)
  line L128 (-0.5, 77.5) -> (-0.5, 62.5)
  line L129 (-0.5, 62.5) -> (-15.5, 62.5)
  line L130 (-40.5, 5.5) -> (-40.5, 20.5)
  line L131 (-40.5, 20.5) -> (-25.5, 20.5)
  line L132 (-25.5, 20.5) -> (-25.5, 5.5)
  line L133 (-25.5, 5.5) -> (-40.5, 5.5)
  line L134 (-58.5, 31.5) -> (-43.5, 31.5)
  line L135 (-43.5, 31.5) -> (-43.5, 16.5)
  line L136 (-43.5, 16.5) -> (-58.5, 16.5)
  line L137 (-58.5, 16.5) -> (-58.5, 31.5)
  line L138 (-22.5, 56.5) -> (-7.5, 56.5)
  line L139 (-7.5, 56.5) -> (-7.5, 41.5)
  line L140 (-7.5, 41.5) -> (-22.5, 41.5)
  line L141 (-22.5, 41.5) -> (-22.5, 56.5)
  line L142 (72.7896, -25.1203) -> (84.2803, -15.4785)
  line L143 (84.2803, -15.4785) -> (93.9221, -26.9691)
  line L144 (93.9221, -26.9691) -> (82.4315, -36.611)
  line L145 (82.4315, -36.611) -> (72.7896, -25.1203)
  line L146 (103.2737, -66.1169) -> (91.783, -75.7587)
  line L147 (91.783, -75.7587) -> (82.1412, -64.2681)
  line L148 (82.1412, -64.2681) -> (93.6319, -54.6263)
  line L149 (93.6319, -54.6263) -> (103.2737, -66.1169)
  line L150 (-33.5, 62.5) -> (-33.5, 77.5)
  line L151 (-33.5, 77.5) -> (-18.5, 77.5)
  line L152 (-18.5, 77.5) -> (-18.5, 62.5)
  line L153 (-18.5, 62.5) -> (-33.5, 62.5)
  line L154 (46.7441, -46.9751) -> (58.2348, -37.3333)
  line L155 (58.2348, -37.3333) -> (67.8766, -48.8239)
  line L156 (67.8766, -48.8239) -> (56.3859, -58.4657)
  line L157 (56.3859, -58.4657) -> (46.7441, -46.9751)
  line L158 (-22.5, 22.5) -> (-7.5, 22.5)
  line L159 (-7.5, 22.5) -> (-7.5, 7.5)
  line L160 (-7.5, 7.5) -> (-22.5, 7.5)
  line L161 (-22.5, 7.5) -> (-22.5, 22.5)
  line L162 (41.1433, 18.8173) -> (52.634, 28.4591)
  line L163 (52.634, 28.4591) -> (62.2758, 16.9684)
  line L164 (62.2758, 16.9684) -> (50.7851, 7.3266)
  line L165 (50.7851, 7.3266) -> (41.1433, 18.8173)
  line L166 (73.9427, 12.3986) -> (64.3009, 23.8893)
  line L167 (64.3009, 23.8893) -> (75.7916, 33.5311)
  line L168 (75.7916, 33.5311) -> (85.4334, 22.0405)
  line L169 (85.4334, 22.0405) -> (73.9427, 12.3986)
  line L170 (-61.5, 52.5) -> (-61.5, 37.5)
  line L171 (-61.5, 37.5) -> (-76.5, 37.5)
  line L172 (-76.5, 37.5) -> (-76.5, 52.5)
  line L173 (-76.5, 52.5) -> (-61.5, 52.5)
  line L174 (-79.5, 49.5) -> (-94.5, 49.5)
  line L175 (-94.5, 49.5) -> (-94.5, 64.5)
  line L176 (-94.5, 64.5) -> (-79.5, 64.5)
  line L177 (-79.5, 64.5) -> (-79.5, 49.5)
  line L178 (-25.5, 54.5) -> (-25.5, 39.5)
  line L179 (-25.5, 39.5) -> (-40.5, 39.5)
  line L180 (-40.5, 39.5) -> (-40.5, 54.5)
  line L181 (-40.5, 54.5) -> (-25.5, 54.5)
  line L182 (-79.5, 47.5) -> (-79.5, 32.5)
  line L183 (-79.5, 32.5) -> (-94.5, 32.5)
  line L184 (-94.5, 32.5) -> (-94.5, 47.5)
  line L185 (-94.5, 47.5) -> (-79.5, 47.5)
  line L186 (-112.5, 19.5) -> (-112.5, 34.5)
  line L187 (-112.5, 34.5) -> (-97.5, 34.5)
  line L188 (-97.5, 34.5) -> (-97.5, 19.5)
  line L189 (-97.5, 19.5) -> (-112.5, 19.5)
  line L190 (36.2303, -4.8864) -> (24.7396, -14.5282)
  line L191 (24.7396, -14.5282) -> (15.0978, -3.0375)
  line L192 (15.0978, -3.0375) -> (26.5884, 6.6043)
  line L193 (26.5884, 6.6043) -> (36.2303, -4.8864)
  line L194 (79.2878, -15.7515) -> (67.7971, -25.3933)
  line L195 (67.7971, -25.3933) -> (58.1553, -13.9026)
  line L196 (58.1553, -13.9026) -> (69.646, -4.2608)
  line L197 (69.646, -4.2608) -> (79.2878, -15.7515)
  line L198 (-58.5, 14.5) -> (-43.5, 14.5)
  line L199 (-43.5, 14.5) -> (-43.5, -0.5)
  line L200 (-43.5, -0.5) -> (-58.5, -0.5)
  line L201 (-58.5, -0.5) -> (-58.5, 14.5)
  line L202 (-76.5, 35.5) -> (-61.5, 35.5)
  line L203 (-61.5, 35.5) -> (-61.5, 20.5)
  line L204 (-61.5, 20.5) -> (-76.5, 20.5)
  line L205 (-76.5, 20.5) -> (-76.5, 35.5)
  line L206 (-112.5, 68.5) -> (-97.5, 68.5)
  line L207 (-97.5, 68.5) -> (-97.5, 53.5)
  line L208 (-97.5, 53.5) -> (-112.5, 53.5)
  line L209 (-112.5, 53.5) -> (-112.5, 68.5)
  line L210 (104.8058, -64.8313) -> (95.164, -53.3407)
  line L211 (95.164, -53.3407) -> (106.6546, -43.6989)
  line L212 (106.6546, -43.6989) -> (116.2964, -55.1895)
  line L213 (116.2964, -55.1895) -> (104.8058, -64.8313)
  line L214 (36.8024, 73.0075) -> (34.478, 68.0228)
  line L215 (34.478, 68.0228) -> (23.9648, 72.9252)
  line L216 (34.478, 68.0228) -> (44.9912, 63.1205)
  line L217 (23.9648, 72.9252) -> (44.9912, 63.1205)
  line L218 (44.9912, 63.1205) -> (40.0888, 52.6073)
  line L219 (40.0888, 52.6073) -> (19.0625, 62.412)
  line L220 (19.0625, 62.412) -> (23.9648, 72.9252)
  dimension "d174" = 5.5
  dimension "d175" = 11.6
  dimension "d176" = 11.6
  dimension "d177" = 11.6
  constraint midpoint L27 L214.start
  constraint perpendicular L27 L214
  constraint perpendicular L214 L215
  constraint perpendicular L214 L216
  constraint perpendicular L217 L218
  constraint parallel L217 L219
  constraint parallel L218 L220
  constraint perpendicular L214 L217
  measures "d174" distance of L214.start L214.end
  measures "d175" distance of L214.end L215.end
  measures "d176" distance of L214.end L216.end
  measures "d177" distance of L215.end L219.end
extrude "Extrude21" cut sketch "Sketch21" against normal blind 2.3 contours L215 L216 L217 L218 L219 L220